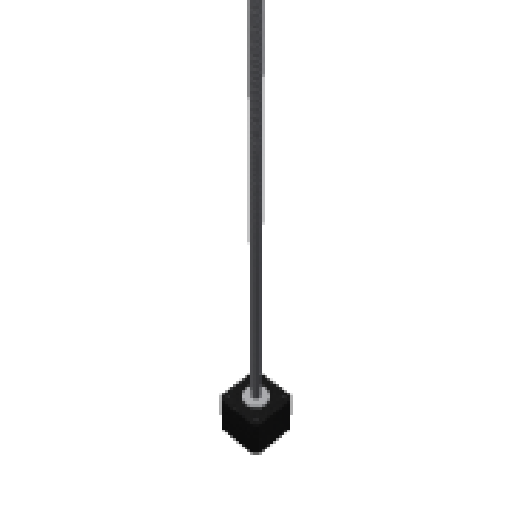
# Autodesk Inventor part: Motor_Z
Saved by Autodesk Inventor 2023.2 (Build 272271000, 271)
## iProperties
Created: 2020-05-09
Part Number: Motor_Z
Material: Steel, Alloy
Document SubType Name: Modeling
Designer: Remo
Mass: 602.679 g
Surface Area: 184.326 cm^2
Volume: 77.9663 cm^3
Density: 7.73 g/cm^3
Appearance: Machined - Aluminum
Author: Remo
Autodesk Inventor part; units mm, degrees
ref_plane "YZ Plane" through (0, 0, 0) normal (1, 0, 0) x (0, 1, 0)
ref_plane "XZ Plane" through (0, 0, 0) normal (0, 1, 0) x (-1, 0, 0)
ref_plane "XY Plane" through (0, 0, 0) normal (0, 0, 1) x (1, 0, 0)
sketch "Sketch1" plane through (0, 0, 0) normal (0, 0, 1) x (1, 0, 0)
  line L0 (21, -21) -> (-21, -21)
  line L1 (-21, -21) -> (-21, 21)
  line L2 (-21, 21) -> (21, 21)
  line L3 (21, 21) -> (21, -21)
  line L4 (21, -21) -> (-21, 21) construction
  line L5 (-21, -21) -> (21, 21) construction
  point P0 (0, 0)
  dimension "d0" = 42
  constraints: 12 end point, 2 midpoint, 2 parallel, 2 perpendicular, 1 horizontal
  measures "d0" distance of L1.end L2.end
extrude "Extrusion1" add sketch "Sketch1" along normal blind 34
chamfer "Chamfer1" distance 3.5 angle 45 4 edges at (-21, 21, 17) (21, 21, 17) (21, -21, 17) (-21, -21, 17)
sketch "Sketch2" plane through (0, 0, 34) normal (0, 0, 1) x (1, 0, 0)
  circle A0 centre (0, 0) radius 11
  dimension "d6" = 22
  constraints: 1 centre point, 1 coincident
  measures "d6" diameter of A0
extrude "Extrusion2" add sketch "Sketch2" along normal blind 2
sketch "Sketch3" plane through (0, 0, 36) normal (0, 0, 1) x (1, 0, 0)
  circle A0 centre (0, 0) radius 4
  dimension "d9" = 8
  constraints: 1 centre point, 1 coincident
  measures "d9" diameter of A0
extrude "Extrusion3" add sketch "Sketch3" along normal blind 300
thread "Thread1" size "M8x1.25" class "6g" standard "ANSI Metric M Profile" full length
chamfer "Chamfer2" distance 1 angle 45 1 edges at (-4, 0, 336)
sketch "Sketch4" plane through (0, 0, 34) normal (0, 0, 1) x (1, 0, 0)
  line L0 (-17.5, -21) -> (17.5, -21) projected
  line L1 (17.5, 21) -> (-17.5, 21) projected
  line L2 (-21, 17.5) -> (-21, -17.5) projected
  point P0 (0, 0)
  point P1 (-15.5, 15.5)
  point P2 (-15.5, -15.5)
  point P3 (15.5, -15.5)
  point P4 (15.5, 15.5)
  dimension "d17" = 31
  dimension "d18" = 31
  dimension "d19" = 42
  dimension "d21" = 5.5
  dimension "d22" = 5.5
  constraints: 2 horizontal alignment, 2 vertical alignment
  measures "d17" distance of point (15.5, 15.5) point (-15.5, 15.5)
  measures "d18" distance of point (-15.5, -15.5) point (-15.5, 15.5)
  measures "d19" distance between parallel lines of L0 L1
  measures "d21" distance from line of L1 point (-15.5, 15.5)
  measures "d22" distance from line of L2 point (-15.5, 15.5)
hole "Hole1" at (-15.5, 15.5, 34) at (-15.5, -15.5, 34) at (15.5, -15.5, 34) at (15.5, 15.5, 34) direction (0, 0, -1) diameter 2.459 depth 8.8 tip angle 118 thread size "M3x0.5" class "6H" standard "ISO Metric profile"
equation "\"d21\" = -0.5 * d18 + 0.5 * d19"
equation "\"d22\" = -0.5 * d18 + 0.5 * d19"
body "Solid1"
